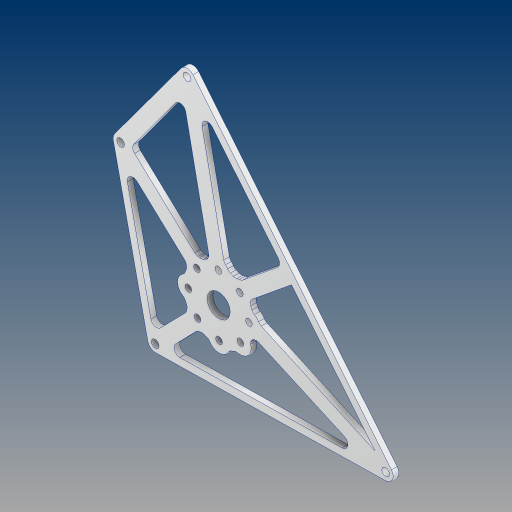
# Autodesk Inventor part: SHOT_1_015_PivotCover
Saved by Autodesk Inventor 2024.3 (Build 283343000, 343)
## iProperties
Created: 2024-08-09
Part Number: SHOT_1_015_PivotCover
Material: Aluminum 6061
Document SubType Name: Modeling
Designer: Kenji
Density: 2.7 g/cm^3
Appearance: Aluminum - Flat
Author: Kenji
Autodesk Inventor part; units mm, degrees
ref_plane "YZ Plane" through (0, 0, 0) normal (1, 0, 0) x (0, 1, 0)
ref_plane "XZ Plane" through (0, 0, 0) normal (0, 1, 0) x (-1, 0, 0)
ref_plane "XY Plane" through (0, 0, 0) normal (0, 0, 1) x (1, 0, 0)
sketch "Sketch2" plane through (0, 0, 0) normal (0, 0, 1) x (1, 0, 0)
  line L0 (0, 0) -> (264.075, 76.1785) construction
  circle A0 centre (264.075, 76.1785) radius 3.2512
  line L1 (0, 0) -> (41.9951, 204.3053) construction
  circle A1 centre (41.9951, 204.3053) radius 3.2512
  line L2 (0, 0) -> (97.7, 279.7575) construction
  circle A2 centre (97.7, 279.7575) radius 3.2512
  line L3 (0, 0) -> (70.949, 72.7241) construction
  circle A3 centre (70.949, 72.7241) radius 3.2512
  circle A4 centre (0, 0) radius 142.24 construction
  circle A5 centre (124.1608, 127.2672) radius 35.56 construction
  circle A6 centre (124.1608, 127.2672) radius 30 construction
  circle A7 centre (97.7, 279.7575) radius 6.35 construction
  circle A8 centre (41.9951, 204.3053) radius 6.35 construction
  circle A9 centre (70.949, 72.7241) radius 6.35 construction
  circle A10 centre (264.075, 76.1785) radius 6.35 construction
  line L4 (102.6169, 283.7758) -> (268.9919, 80.1968)
  line L5 (71.0626, 66.3751) -> (264.1886, 69.8295)
  line L6 (64.7474, 71.3595) -> (35.7934, 202.9407)
  line L7 (36.8865, 208.0769) -> (92.5914, 283.5291)
  arc A11 (36.8865, 208.0769) -> (35.7934, 202.9407) centre (41.9951, 204.3053) ccw
  arc A12 (102.6169, 283.7758) -> (92.5914, 283.5291) centre (97.7, 279.7575) ccw
  arc A13 (264.1886, 69.8295) -> (268.9919, 80.1968) centre (264.075, 76.1785) ccw
  arc A14 (64.7474, 71.3595) -> (71.0626, 66.3751) centre (70.949, 72.7241) ccw
  circle A15 centre (124.1608, 127.2672) radius 25.4 construction
  circle A16 centre (141.898, 145.4482) radius 2.794
  circle A17 centre (123.847, 152.6653) radius 2.794
  circle A18 centre (105.9798, 145.0045) radius 2.794
  circle A19 centre (98.7627, 126.9534) radius 2.794
  circle A20 centre (106.4235, 109.0862) radius 2.794
  circle A21 centre (124.4746, 101.8691) radius 2.794
  circle A22 centre (142.3418, 109.5299) radius 2.794
  circle A23 centre (149.5588, 127.581) radius 2.794
  circle A24 centre (124.1608, 127.2672) radius 9.652
  dimension "d84" = 50.8
  dimension "d63" = 6.5024
  dimension "d64" = 274.8432
  dimension "d65" = 76.1785
  dimension "d66" = 208.5767
  dimension "d67" = 6.5024
  dimension "d68" = 204.3053
  dimension "d69" = 6.5024
  dimension "d70" = 296.3268
  dimension "d71" = 279.7575
  dimension "d72" = 101.6
  dimension "d73" = 6.5024
  dimension "d74" = 72.7241
  dimension "d75" = 284.48
  dimension "d76" = 71.12
  dimension "d77" = 60
  dimension "d78" = 12.7
  dimension "d79" = 12.7
  dimension "d80" = 12.7
  dimension "d81" = 12.7
  dimension "d85" = 5.588
  dimension "d88" = 360
  dimension "d142" = 19.304
  constraints: 24 centre point, 17 point on circle, 16 end point, 12 coincident, 11 tangent, 3 concentric, 2 point on line, 21 other
  measures "d63" diameter of A0
  measures "d64" distance of L0.start L0.end
  measures "d65" vertical distance of L0.start L0.end
  measures "d66" distance of L0.start L1.end
  measures "d67" diameter of A1
  measures "d68" vertical distance of L0.start L1.end
  measures "d69" diameter of A2
  measures "d70" distance of L0.start L2.end
  measures "d71" vertical distance of L0.start L2.end
  measures "d72" distance of L0.start L3.end
  measures "d73" diameter of A3
  measures "d74" vertical distance of L0.start L3.end
  measures "d75" diameter of A4
  measures "d76" diameter of A5
  measures "d77" diameter of A6
  measures "d78" diameter of A7
  measures "d79" diameter of A8
  measures "d80" diameter of A9
  measures "d81" diameter of A10
  measures "d85" diameter of A16
  measures "d142" diameter of A24
extrude "Extrusion5" add sketch "Sketch2" against normal blind 4.7625
sketch "Sketch4" plane through (0, 0, 0) normal (0, 0, 1) x (1, 0, 0)
  line L0 (35.7934, 202.9407) -> (64.7474, 71.3595) construction
  arc A0 (64.7474, 71.3595) -> (71.0626, 66.3751) centre (70.949, 72.7241) ccw construction
  line L1 (71.0626, 66.3751) -> (264.1886, 69.8295) construction
  arc A1 (264.1886, 69.8295) -> (268.9919, 80.1968) centre (264.075, 76.1785) ccw construction
  line L2 (268.9919, 80.1968) -> (102.6169, 283.7758) construction
  arc A2 (102.6169, 283.7758) -> (92.5914, 283.5291) centre (97.7, 279.7575) ccw construction
  line L3 (92.5914, 283.5291) -> (36.8865, 208.0769) construction
  arc A3 (36.8865, 208.0769) -> (35.7934, 202.9407) centre (41.9951, 204.3053) ccw construction
  circle A4 centre (97.7, 279.7575) radius 3.2512 construction
  circle A5 centre (98.7627, 126.9534) radius 2.794 construction
  circle A6 centre (124.1608, 127.2672) radius 9.652 construction
  circle A7 centre (149.5588, 127.581) radius 2.794 construction
  circle A8 centre (142.3418, 109.5299) radius 2.794 construction
  circle A9 centre (124.4746, 101.8691) radius 2.794 construction
  circle A10 centre (106.4235, 109.0862) radius 2.794 construction
  circle A11 centre (105.9798, 145.0045) radius 2.794 construction
  circle A12 centre (123.847, 152.6653) radius 2.794 construction
  circle A13 centre (141.898, 145.4482) radius 2.794 construction
  circle A14 centre (70.949, 72.7241) radius 3.2512 construction
  circle A15 centre (41.9951, 204.3053) radius 3.2512 construction
  circle A16 centre (264.075, 76.1785) radius 3.2512 construction
  circle A17 centre (41.9951, 204.3053) radius 9.6012 construction
  circle A18 centre (70.949, 72.7241) radius 9.6012 construction
  circle A19 centre (124.1608, 127.2672) radius 16.002 construction
  circle A20 centre (98.7627, 126.9534) radius 9.144 construction
  circle A21 centre (105.9798, 145.0045) radius 9.144 construction
  circle A22 centre (106.4235, 109.0862) radius 9.144 construction
  circle A23 centre (124.4746, 101.8691) radius 9.144 construction
  circle A24 centre (142.3418, 109.5299) radius 9.144 construction
  circle A25 centre (149.5588, 127.581) radius 9.144 construction
  circle A26 centre (141.898, 145.4482) radius 9.144 construction
  circle A27 centre (123.847, 152.6653) radius 9.144 construction
  circle A28 centre (97.7, 279.7575) radius 9.6012 construction
  circle A29 centre (264.075, 76.1785) radius 9.6012 construction
  line L4 (97.7, 279.7575) -> (264.075, 76.1785) construction
  line L5 (264.075, 76.1785) -> (70.949, 72.7241) construction
  line L6 (70.949, 72.7241) -> (41.9951, 204.3053) construction
  line L7 (41.9951, 204.3053) -> (97.7, 279.7575) construction
  line L8 (97.7, 279.7575) -> (123.847, 152.6653) construction
  line L9 (123.847, 152.6653) -> (105.9798, 145.0045) construction
  line L10 (105.9798, 145.0045) -> (41.9951, 204.3053) construction
  line L11 (115.7983, 160.2758) -> (96.5081, 254.0391)
  line L12 (87.9892, 255.9131) -> (53.0131, 208.5381)
  line L13 (53.6088, 202.1995) -> (104.1609, 155.348)
  line L14 (111.1656, 154.137) -> (113.0028, 154.9247)
  arc A30 (96.5081, 254.0391) -> (87.9892, 255.9131) centre (91.8309, 253.0769) ccw
  arc A31 (53.0131, 208.5381) -> (53.6088, 202.1995) centre (56.8548, 205.7018) ccw
  arc A32 (108.1503, 153.8871) -> (106.9173, 154.1003) centre (105.9798, 145.0045) ccw
  arc A33 (116.3014, 157.8302) -> (115.2975, 155.9086) centre (123.847, 152.6653) ccw construction
  arc A34 (113.0028, 154.9247) -> (115.7983, 160.2758) centre (111.121, 159.3135) ccw
  arc A35 (108.1503, 153.8871) -> (111.1656, 154.137) centre (109.2838, 158.5258) ccw
  arc A36 (104.1609, 155.348) -> (106.9173, 154.1003) centre (107.4069, 158.8503) ccw
  line L15 (148.9783, 151.2346) -> (181.2088, 177.5749) construction
  line L16 (132.3375, 149.2706) -> (133.4075, 148.8428) construction
  line L17 (133.9716, 155.456) -> (136.4882, 154.4499)
  line L18 (144.3569, 155.6585) -> (173.493, 179.47)
  line L19 (128.3811, 162.1383) -> (110.277, 250.1367)
  arc A37 (131.6628, 157.4114) -> (129.8982, 159.5206) centre (123.847, 152.6653) ccw
  arc A38 (141.5282, 154.5847) -> (139.5087, 154.2745) centre (141.898, 145.4482) ccw
  line L20 (174.1687, 186.1893) -> (118.6517, 254.1207)
  arc A39 (118.6517, 254.1207) -> (110.277, 250.1367) centre (114.9542, 251.0989) ccw
  arc A40 (173.493, 179.47) -> (174.1687, 186.1893) centre (170.4712, 183.1675) ccw
  arc A41 (141.5282, 154.5847) -> (144.3569, 155.6585) centre (141.3351, 159.356) ccw
  arc A42 (136.4882, 154.4499) -> (139.5087, 154.2745) centre (138.2609, 158.8838) ccw
  arc A43 (131.6628, 157.4114) -> (133.9716, 155.456) centre (135.7444, 159.89) ccw
  arc A44 (128.3811, 162.1383) -> (129.8982, 159.5206) centre (133.0583, 163.1006) ccw
  line L21 (157.901, 123.8365) -> (255.3158, 80.1103) construction
  line L22 (145.5014, 137.0441) -> (145.9555, 135.9851) construction
  line L23 (152.4019, 145.8317) -> (185.2271, 172.6581)
  line L24 (151.0349, 140.2524) -> (152.0986, 137.7715)
  line L25 (159.7907, 129.9486) -> (255.091, 87.1715)
  line L26 (185.2271, 172.6581) -> (255.091, 87.1715)
  arc A45 (150.327, 141.9034) -> (151.011, 144.6949) centre (141.898, 145.4482) ccw construction
  arc A46 (157.5651, 131.9983) -> (154.1105, 135.5117) centre (149.5588, 127.581) ccw
  arc A47 (152.0986, 137.7715) -> (154.1105, 135.5117) centre (156.4874, 139.6532) ccw
  arc A48 (157.5651, 131.9983) -> (159.7907, 129.9486) centre (161.7462, 134.3051) ccw
  arc A49 (152.4019, 145.8317) -> (151.0349, 140.2524) centre (155.4237, 142.1342) ccw
  line L27 (77.6537, 79.5965) -> (100.0381, 102.541) construction
  line L28 (114.9141, 105.6915) -> (115.984, 105.2638) construction
  line L29 (133.9377, 105.9266) -> (132.8787, 105.4725) construction
  line L30 (146.1642, 119.0905) -> (145.7364, 118.0205) construction
  line L31 (88.0917, 81.2024) -> (105.1273, 98.6642)
  line L32 (111.8334, 100.0845) -> (114.3499, 99.0784)
  line L33 (137.156, 100.3974) -> (134.6651, 99.3294)
  line L34 (151.1496, 114.4549) -> (151.0318, 114.1602)
  line L35 (157.539, 117.0386) -> (229.6718, 84.6606)
  line L36 (227.8018, 75.5297) -> (91.5952, 73.0934)
  arc A50 (80.5487, 72.8958) -> (80.5232, 73.4445) centre (70.949, 72.7241) ccw
  arc A51 (107.8174, 100.049) -> (108.8129, 100.2599) centre (106.4235, 109.0862) ccw
  arc A52 (116.6588, 97.123) -> (132.4053, 97.3175) centre (124.4746, 101.8691) ccw
  arc A53 (140.1713, 100.6473) -> (150.9905, 112.4987) centre (142.3418, 109.5299) ccw
  arc A54 (157.539, 117.0386) -> (151.1496, 114.4549) centre (155.5835, 112.6821) ccw
  circle A55 centre (153.2487, 113.2738) radius 2.3876 construction
  arc A56 (151.0318, 114.1602) -> (150.9905, 112.4987) centre (153.2487, 113.2738) ccw
  arc A57 (140.1713, 100.6473) -> (137.156, 100.3974) centre (139.0377, 96.0086) ccw
  arc A58 (134.6651, 99.3294) -> (132.4053, 97.3175) centre (136.5468, 94.9406) ccw
  arc A59 (116.6588, 97.123) -> (114.3499, 99.0784) centre (112.5772, 94.6444) ccw
  arc A60 (111.8334, 100.0845) -> (108.8129, 100.2599) centre (110.0607, 95.6506) ccw
  arc A61 (107.8174, 100.049) -> (105.1273, 98.6642) centre (108.5454, 95.3296) ccw
  arc A62 (88.0917, 81.2024) -> (91.5952, 73.0934) centre (91.5098, 77.8678) ccw
  arc A63 (227.8018, 75.5297) -> (229.6718, 84.6606) centre (227.7164, 80.3041) ccw
  line L37 (102.5851, 136.5139) -> (102.1573, 135.4439) construction
  line L38 (102.3661, 118.5493) -> (102.8202, 117.4902) construction
  line L39 (96.223, 116.7629) -> (97.291, 114.272)
  line L40 (96.9781, 139.5946) -> (95.972, 137.078)
  line L41 (75.4962, 86.4783) -> (96.0368, 107.5329)
  arc A64 (97.5409, 111.2567) -> (97.3547, 110.2564) centre (106.4235, 109.0862) ccw
  arc A65 (94.0166, 134.7692) -> (94.2111, 119.0227) centre (98.7627, 126.9534) ccw
  line L42 (95.5281, 146.0333) -> (55.5759, 183.0608)
  line L43 (47.6663, 178.5323) -> (67.4145, 88.7867)
  arc A66 (67.4145, 88.7867) -> (75.4962, 86.4783) centre (72.0781, 89.8129) ccw
  arc A67 (96.0368, 107.5329) -> (97.3547, 110.2564) centre (92.6188, 110.8675) ccw
  arc A68 (97.5409, 111.2567) -> (97.291, 114.272) centre (92.9022, 112.3902) ccw
  arc A69 (96.223, 116.7629) -> (94.2111, 119.0227) centre (91.8342, 114.8812) ccw
  arc A70 (94.0166, 134.7692) -> (95.972, 137.078) centre (91.538, 138.8508) ccw
  arc A71 (96.9813, 143.3795) -> (97.1534, 142.6151) centre (105.9798, 145.0045) ccw
  arc A72 (96.9813, 143.3795) -> (95.5281, 146.0333) centre (92.2821, 142.5309) ccw
  arc A73 (96.9781, 139.5946) -> (97.1534, 142.6151) centre (92.5442, 141.3673) ccw
  arc A74 (55.5759, 183.0608) -> (47.6663, 178.5323) centre (52.33, 179.5585) ccw
  point P0 (0, 0)
  point P1 (105.4705, 154.1343)
  point P2 (109.5245, 153.4334)
  point P3 (132.3137, 156.1189)
  point P4 (138.1461, 153.787)
  point P5 (142.9743, 154.5287)
  point P6 (177.1904, 182.4918)
  point P7 (128.7409, 160.3894)
  point P8 (106.3641, 269.156)
  point P9 (152.8022, 136.1304)
  point P10 (158.1618, 130.6798)
  point P11 (106.3742, 99.9423)
  point P12 (110.1755, 100.7474)
  point P13 (116.0079, 98.4155)
  point P14 (138.797, 101.101)
  point P15 (133.024, 98.6258)
  point P16 (249.1627, 75.9118)
  point P17 (95.5193, 118.4039)
  point P18 (97.9946, 112.631)
  point P19 (97.641, 141.2525)
  point P20 (95.3091, 135.4201)
  point P21 (71.4326, 82.3131)
  point P22 (97.2837, 108.8109)
  point P23 (96.8376, 144.8195)
  point P24 (44.3882, 193.4295)
  point P25 (68.8857, 82.101)
  dimension "d145" = 6.35
  dimension "d146" = 6.35
  dimension "d147" = 6.35
  dimension "d148" = 6.35
  dimension "d149" = 6.35
  dimension "d150" = 6.35
  dimension "d151" = 6.35
  dimension "d152" = 6.35
  dimension "d153" = 6.35
  dimension "d154" = 6.35
  dimension "d155" = 6.35
  dimension "d156" = 6.35
  dimension "d157" = 6.35
  dimension "d158" = 6.35
  dimension "d159" = 6.35
  dimension "d160" = 4.7752
  dimension "d161" = 4.7752
  dimension "d162" = 6.35
  dimension "d163" = 6.35
  dimension "d164" = 6.35
  dimension "d165" = 4.7752
  dimension "d166" = 6.35
  dimension "d167" = 6.35
  dimension "d168" = 6.35
  dimension "d169" = 4.7752
  dimension "d170" = 6.35
  dimension "d171" = 6.35
  dimension "d172" = 6.35
  dimension "d173" = 6.35
  dimension "d174" = 6.35
  dimension "d175" = 4.7752
  dimension "d176" = 4.7752
  dimension "d177" = 4.7752
  dimension "d178" = 4.7752
  dimension "d179" = 6.35
  dimension "d180" = 6.35
  dimension "d181" = 6.35
  dimension "d182" = 6.35
  dimension "d183" = 4.7752
  dimension "d184" = 4.7752
  dimension "d185" = 4.7752
  constraints: 141 point on circle, 80 end point, 64 point on line, 62 tangent, 55 centre point, 20 equal radius, 14 parallel, 10 concentric, 1 collinear, 1 perpendicular, 31 other
  measures "d145" radial gap between concentric circles of A15 A17
  measures "d146" radial gap between concentric circles of A14 A18
  measures "d147" radial gap between concentric circles of A6 A19
  measures "d148" radial gap between concentric circles of A5 A20
  measures "d149" radial gap between concentric circles of A11 A21
  measures "d151" radial gap between concentric circles of A9 A23
  measures "d152" radial gap between concentric circles of A8 A24
  measures "d153" radial gap between concentric circles of A7 A25
  measures "d155" radial gap between concentric circles of A12 A27
  measures "d156" radial gap between concentric circles of A4 A28
  measures "d158" distance between parallel lines of L2 L4
  measures "d159" distance between parallel lines of L8 L11
  measures "d160" radius of A30
  measures "d161" radius of A34
  measures "d162" distance between parallel lines of L16 L17
  measures "d163" distance between parallel lines of L15 L18
  measures "d164" distance between parallel lines of L8 L19
  measures "d165" radius of A39
  measures "d166" distance between parallel lines of L15 L23
  measures "d167" distance between parallel lines of L22 L24
  measures "d168" distance between parallel lines of L21 L25
  measures "d169" radius of A47
  measures "d170" distance between parallel lines of L27 L31
  measures "d171" distance between parallel lines of L28 L32
  measures "d172" distance between parallel lines of L29 L33
  measures "d173" distance between parallel lines of L30 L34
  measures "d174" distance between parallel lines of L21 L35
  measures "d175" radius of A54
  measures "d176" diameter of A55
  measures "d177" radius of A57
  measures "d178" radius of A62
  measures "d179" distance between parallel lines of L38 L39
  measures "d180" distance between parallel lines of L37 L40
  measures "d181" distance between parallel lines of L27 L41
  measures "d182" distance between parallel lines of L10 L42
  measures "d183" radius of A66
  measures "d184" radius of A72
  measures "d185" radius of A74
extrude "Extrusion6" cut sketch "Sketch4" against normal blind 4.7625
body "Solid4"
